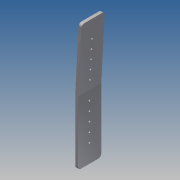
# Autodesk Inventor part: joinerBracket
Saved by Autodesk Inventor 2014 SP1 (Build 180222100, 222)
## iProperties
Created: 2014-09-15
Part Number: joinerBracket
Material: Steel
Document SubType Name: Sheet Metal
Designer: Dave
Mass: 115.602 g
Surface Area: 125.495 cm^2
Volume: 14.7264 cm^3
Density: 7.85 g/cm^3
Appearance: Steel
Sheet Metal Rule: Default
Author: Dave
Autodesk Inventor part; units mm, degrees
ref_plane "YZ Plane" through (0, 0, 0) normal (1, 0, 0) x (0, 1, 0)
ref_plane "XZ Plane" through (0, 0, 0) normal (0, 1, 0) x (-1, 0, 0)
ref_plane "XY Plane" through (0, 0, 0) normal (0, 0, 1) x (1, 0, 0)
sketch "Sketch1" plane through (0, 0, 0) normal (1, 0, 0) x (0, 1, 0)
  line L0 (3.175, 0) -> (136.825, 0)
  line L1 (140, -3.175) -> (140, -22.225)
  line L2 (136.825, -25.4) -> (3.175, -25.4)
  line L3 (0, -22.225) -> (0, -3.175)
  arc A0 (140, -3.175) -> (136.825, 0) centre (136.825, -3.175) ccw
  arc A1 (136.825, -25.4) -> (140, -22.225) centre (136.825, -22.225) ccw
  arc A2 (0, -22.225) -> (3.175, -25.4) centre (3.175, -22.225) ccw
  arc A3 (3.175, 0) -> (0, -3.175) centre (3.175, -3.175) ccw
  point P0 (0, 0)
  point P1 (140, 0)
  point P2 (0, -25.4)
  dimension "d0" = 25.4
  dimension "d1" = 140
  dimension "d2" = 3.175
  constraints: 8 end point, 8 point on circle, 8 tangent, 6 point on line, 4 centre point, 3 equal radius, 2 parallel, 1 horizontal, 1 perpendicular
  measures "d0" distance of point (0, -25.4) point (0, 0)
  measures "d1" distance of point (0, 0) point (140, 0)
  measures "d2" radius of A0
extrude "Extrusion1" add sketch "Sketch1" along normal blind 3.048
sketch "Sketch3" plane through (3.048, 0, 0) normal (1, 0, 0) x (0, 0, -1)
  line L0 (22.225, 140) -> (3.175, 140) projected
  line L1 (0, 136.825) -> (0, 3.175) projected
  circle A0 centre (12.7, 120) radius 1.9226
  circle A1 centre (12.7, 100) radius 1.9226
  circle A2 centre (12.7, 80) radius 1.9226
  circle A3 centre (12.7, 60) radius 1.9226
  circle A4 centre (12.7, 40) radius 1.9226
  circle A5 centre (12.7, 20) radius 1.9226
  point P0 (0, 0)
  dimension "d29" = 20
  dimension "d32" = 20
  constraints: 6 centre point, 1 vertical, 10 other
  measures "d29" distance from line of A0.centre L0
  measures "d32" distance of A0.centre A1.centre
hole "Hole2" at (3.048, 40, -12.7) at (3.048, 20, -12.7) at (3.048, 60, -12.7) at (3.048, 80, -12.7) at (3.048, 100, -12.7) at (3.048, 120, -12.7) direction (-1, 0, 0) diameter 2 depth 25.4 tip angle 118
sketch "Sketch4" plane through (3.048, 0, 0) normal (1, 0, 0) x (0, 0, -1)
  line L0 (0, 136.825) -> (0, 3.175) projected
  line L1 (25.4, 3.175) -> (25.4, 136.825) projected
  line L2 (0, 70) -> (25.4, 70) construction
  point P0 (0, 0)
  constraints: 2 end point, 2 midpoint
fold "Fold1" angle 3.2 bend radius 3.048 thickness 3.048 k factor 0.44 line from (3.048, 70, 0) to (3.048, 70, -25.4) line at bend centre moving side (0, 1, 0) folds toward (1, 0, 0)
sketch "Sketch5" plane through (3.0528, 70.0476, 0) normal (0.9984408, -0.0558215, 0) x (0, 0, -1)
  line L0 (25.4, 0) -> (25.4, 66.7024) projected
  circle A0 centre (12.7, 49.8774) radius 1 projected
  circle A1 centre (12.7, 39.8774) radius 1.2396
  circle A2 centre (12.7, 19.8774) radius 1.2396
  point P0 (0, -70.1088)
  dimension "d50" = 10
  dimension "d53" = 20
  constraints: 2 centre point, 1 vertical, 2 other
  measures "d50" distance of A1.centre A0.centre
  measures "d53" distance of A1.centre A2.centre
hole "Hole3" at (5.2788, 109.8628, -12.7) at (4.1623, 89.894, -12.7) direction (-0.9984408, 0.0558215, 0) diameter 2 end through all
sketch "Sketch6" plane through (3.048, 0, 0) normal (1, 0, 0) x (0, 0, -1)
  line L0 (0, 69.8774) -> (0, 3.175) projected
  circle A0 centre (12.7, 20) radius 1 projected
  circle A1 centre (12.7, 30) radius 1.1584
  circle A2 centre (12.7, 50) radius 1.1584
  point P0 (0, 0)
  dimension "d65" = 10
  dimension "d68" = 20
  constraints: 2 centre point, 1 vertical, 2 other
  measures "d65" distance of A1.centre A0.centre
  measures "d68" distance of A1.centre A2.centre
hole "Hole4" at (3.048, 50, -12.7) at (3.048, 30, -12.7) direction (-1, 0, 0) diameter 2 end through all
equation "\"d3\" = Thickness"
equation "\"d44\" = BendReliefWidth"
equation "\"d45\" = BendReliefDepth"
equation "\"d46\" = MinimumRemnant"
equation "\"d47\" = BendRadius"
equation "\"d49\" = BendRadius"
equation "\"d63\" = Thickness"
equation "\"d78\" = Thickness"
equation "\"BendRadius\" = Thickness"
equation "\"BendReliefWidth\" = Thickness"
equation "\"BendReliefDepth\" = 0.5 * Thickness"
equation "\"CornerReliefSize\" = 4 * Thickness"
equation "\"MinimumRemnant\" = 2 * Thickness"
equation "\"TransitionRadius\" = BendRadius"
equation "\"JacobiRadiusSize\" = Thickness"
equation "\"GapSize\" = Thickness"
equation "\"Thickness\" = 3.048"
body "Solid1"
